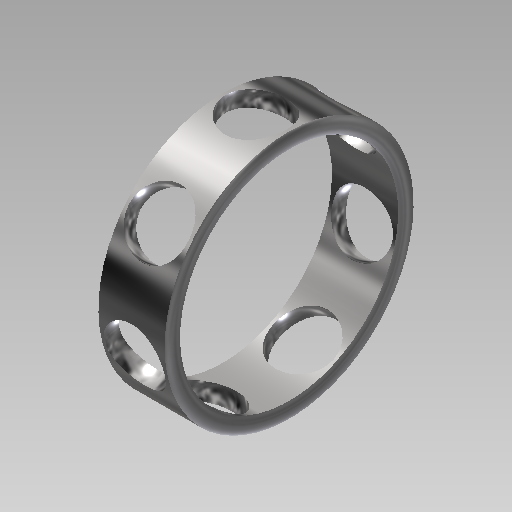
# Autodesk Inventor part: RF-1560ZZ_cage
Saved by Autodesk Inventor 2020 (Build 240168000, 168)
## iProperties
Created: 2019-10-06
Part Number: RF-1560ZZ_cage
Material: 鋼、炭素鋼
Catalog Web Link: www.cadenas.de
Description: Radial Flanged Ball Bearings (RF-Series/LF series) Metric ST cage-Radial Flanged Ball Bearings (RF-Series/LF series) Metric Shielded Type
Vendor: NMB
Document SubType Name: Modeling
Designer: psadmin
Manufacturer: NMB
Mass: 0.313504 g
Surface Area: 2.02725 cm^2
Volume: 0.0399368 cm^3
Density: 7.85 g/cm^3
Appearance: 半つや出し
Category: PARTsolutions
Company: NMB
PSOL_IDENT_0: {$CADENAS_DATA\23d-libs\nmb\pbbp\radial_flanged_ball_bearings\rfbb_rflfs_m\rflf_shielded_cage.prj},2
PSOL_IDENT_1: 29 {VTYP=3D},{NB=RF-1560ZZ_cage},{LINA=RF-1560ZZ_cage},{NN=Radial Flanged Ball Bearings (RF-Series/L
PSOL_IDENT_2: F series) Metric ST cage},{DATE=11.11.2013 05:13:45},{GEOMDATE=24.10.2013 10:21:00},{VERSION=},{LINE
PSOL_IDENT_3: ID=1490},{WBVAR=},{WBNUMERIC=}  {NB=RF-1560ZZ_cage},{LINA=RF-1560ZZ_cage},{KT=DUMMY},{IDNR=},{PN=RF-
PSOL_IDENT_4: 1560ZZ},{SHLD=shielded},{FLANG=flanged},{SD=6.000},{D=15.000},{B=5.000},{SR=0.20},{BCZ=7},{DW=2.7781
PSOL_IDENT_5: },{LI=7.80},{LO=13.20},{D1=17.000},{C1=1.20},{D2=0.0},{C2=0.00},{COR=671},{CR=1058},{PCD=10.500},{U=
PSOL_IDENT_6: 13.278},{W=7.722},{Y=1.389},{Z=1.389},{AA=13.000},{AC=1.00},{AD=0.000},{AF=0.00},{AQ=0.20},{AH=13.40
PSOL_IDENT_7: },{AI=8.00},{AJ=0.40}
NN: Radial Flanged Ball Bearings (RF-Series/LF series) Metric ST cage
NT: Radial Flanged Ball Bearings (RF-Series/LF series) Metric Shielded Type
NB: RF-1560ZZ_cage
NBSYN: $PN._cage
LINA: RF-1560ZZ_cage
PN: RF-1560ZZ
SHLD: shielded
FLANG: flanged
SD: 6
D: 15
B: 5
SR: 0.2
BCZ: 7
DW: 2.7781
LI: 7.8
LO: 13.2
D1: 17
C1: 1.2
D2: 0
C2: 0
COR: 671
CR: 1058
PCD: 10.5
U: 13.278
W: 7.722
Y: 1.389
Z: 1.389
AA: 13
AC: 1
AD: 0
AF: 0
AQ: 0.2
AH: 13.4
AI: 8
AJ: 0.4
SUPPLIER: NMB
ARTICLENO: RF-1560ZZ_cage
BOMINFO: RF-1560ZZ_cage
CREATOR: CADENAS GmbH
Title: RF-1560ZZ_cage
Author: Cadenas PARTsolutions
Comments: Radial Flanged Ball Bearings (RF-Series/LF series) Metric Shielded Type
Autodesk Inventor part; units mm, degrees
note: some values were not read from the file. Chosen so that the rebuilt part matches the saved one: pattern direction of "Circular Pattern1".
sketch "Sketch_6" plane through (0, 0, 0) normal (0, 0, 1) x (1, 0, 0)
  line L0 (3.988, 0) -> (1.012, 0)
  arc A0 (1.012, 5.5973) -> (1.012, 4.9027) centre (2.5, 5.25) ccw
  line L1 (1.012, 4.9027) -> (3.988, 4.9027)
  arc A1 (3.988, 4.9027) -> (3.988, 5.5973) centre (2.5, 5.25) ccw
  line L2 (3.988, 5.5973) -> (1.012, 5.5973)
  constraints: 6 end point, 4 point on circle, 2 centre point
revolve "Revolution1" add sketch "Sketch_6" angle 360 about axis through (3.988, 0, 0) along (1, 0, 0)
sketch "Sketch_2" plane through (2.5, 0, 0) normal (1, 0, 0) x (0, 0, -1)
  line L0 (1.4029, 5.25) -> (-1.4029, 5.25)
  arc A0 (1.4029, 5.25) -> (-1.4029, 5.25) centre (0, 5.25) ccw
  line L1 (1.4029, 5.25) -> (-1.4029, 5.25)
  constraints: 4 end point, 2 point on circle, 1 centre point
revolve "Revolution2" cut sketch "Sketch_2" angle 360 about axis through (2.5, 5.25, -1.4029) along (0, 0, -1)
pattern_circular "Circular Pattern1" count 7 over 360 about axis through (2.5, 0, 0) along (1, 0, 0) of "Revolution2"
ref_plane "1_XY" through (2.5, 0, 0) normal (1, 0, 0) x (0, 0, -1)
ref_plane "1_YZ" through (2.5, 0, 0) normal (0, 0, -1) x (0, 1, 0)
ref_plane "1_ZX" through (2.5, 0, 0) normal (0, 1, 0) x (1, 0, 0)
ref_plane "2_1_XY" through (2.5, 5.25, 0) normal (1, 0, 0) x (0, 0, -1)
ref_plane "2_1_YZ" through (2.5, 5.25, 0) normal (0, 0, -1) x (0, 1, 0)
ref_plane "2_1_ZX" through (2.5, 5.25, 0) normal (0, 1, 0) x (1, 0, 0)
ref_plane "2_2_XY" through (2.5, 3.2733, 4.1046) normal (1, 0, 0) x (0, 0, -1)
ref_plane "2_2_YZ" through (2.5, 3.2733, 4.1046) normal (0, 0, -1) x (0, 1, 0)
ref_plane "2_2_ZX" through (2.5, 3.2733, 4.1046) normal (0, 1, 0) x (1, 0, 0)
ref_plane "2_3_XY" through (2.5, -1.1682, 5.1184) normal (1, 0, 0) x (0, 0, -1)
ref_plane "2_3_YZ" through (2.5, -1.1682, 5.1184) normal (0, 0, -1) x (0, 1, 0)
ref_plane "2_3_ZX" through (2.5, -1.1682, 5.1184) normal (0, 1, 0) x (1, 0, 0)
ref_plane "2_4_XY" through (2.5, -4.7301, 2.2779) normal (1, 0, 0) x (0, 0, -1)
ref_plane "2_4_YZ" through (2.5, -4.7301, 2.2779) normal (0, 0, -1) x (0, 1, 0)
ref_plane "2_4_ZX" through (2.5, -4.7301, 2.2779) normal (0, 1, 0) x (1, 0, 0)
ref_plane "2_5_XY" through (2.5, -4.7301, -2.2779) normal (1, 0, 0) x (0, 0, -1)
ref_plane "2_5_YZ" through (2.5, -4.7301, -2.2779) normal (0, 0, -1) x (0, 1, 0)
ref_plane "2_5_ZX" through (2.5, -4.7301, -2.2779) normal (0, 1, 0) x (1, 0, 0)
ref_plane "2_6_XY" through (2.5, -1.1682, -5.1184) normal (1, 0, 0) x (0, 0, -1)
ref_plane "2_6_YZ" through (2.5, -1.1682, -5.1184) normal (0, 0, -1) x (0, 1, 0)
ref_plane "2_6_ZX" through (2.5, -1.1682, -5.1184) normal (0, 1, 0) x (1, 0, 0)
ref_plane "2_7_XY" through (2.5, 3.2733, -4.1046) normal (1, 0, 0) x (0, 0, -1)
ref_plane "2_7_YZ" through (2.5, 3.2733, -4.1046) normal (0, 0, -1) x (0, 1, 0)
ref_plane "2_7_ZX" through (2.5, 3.2733, -4.1046) normal (0, 1, 0) x (1, 0, 0)
body "Solid1"
